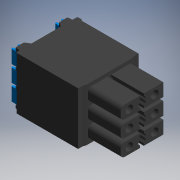
# Autodesk Inventor part: 3943136 6GD-2RR3,5-CLP-CBL
Saved by Autodesk Inventor 2017.3 (Build 213256000, 256)
## iProperties
Part Number: 3943136 6GD-2RR3,5-CLP-CBL
Material: Generic
Catalog Web Link: www.cadenas.de
Description: NEKM-C6 (p)-Terminal strip
Vendor: FESTO
Document SubType Name: Modeling
Designer: partserver
Manufacturer: FESTO
Mass: 2.36353 g
Surface Area: 19.1193 cm^2
Volume: 2.36353 cm^3
Density: 1 g/cm^3
Appearance: PSOLRGB-80-80-80
Category: PARTsolutions
Company: FESTO
Title: 3943136 6GD-2RR3,5-CLP-CBL
Author: Cadenas PARTsolutions
Comments: Terminal strip
PSOL_IDENT_0: {$CADENAS_DATA\23d-libs\festo\parts\n\nekm\parts\nekm_c6_parts.prj},197 {VTYP=3D},{NB=3943136 6GD-2R
PSOL_IDENT_1: R3,5-CLP-CBL},{LINA=3943136 6GD-2RR3,5-CLP-CBL},{NN=NEKM-C6 (p)},{DATE=16.05.2019 05:36:58},{GEOMDAT
PSOL_IDENT_2: E=16.05.2019 05:36:56},{VERSION=},{LINEID=10},{WBVAR=},{WBNUMERIC=}  {NB=3943136 6GD-2RR3,5-CLP-CBL}
PSOL_IDENT_3: ,{LINA=3943136 6GD-2RR3,5-CLP-CBL},{KT=DUMMY},{TNR=3943136},{TYP=6GD-2RR3,5-CLP-CBL},{VERS=1},{N=3},
PSOL_IDENT_4: {L=11.300},{L1=0.000}
NB: 3943136 6GD-2RR3,5-CLP-CBL
NN: NEKM-C6 (p)
NT: Terminal strip
NBSYN: $TNR. $TYP.
LINA: 3943136 6GD-2RR3,5-CLP-CBL
CATALOG: Festo
TNR: 3943136
TYP: 6GD-2RR3,5-CLP-CBL
VERS: 1
N: 3
L: 11.3
L1: 0
SUPPLIER: FESTO
ARTICLENO: 3943136 6GD-2RR3,5-CLP-CBL
BOMINFO: 3943136 6GD-2RR3,5-CLP-CBL
CREATOR: CADENAS GmbH
Autodesk Inventor part; units mm, degrees
sketch "Sketch_1" plane through (0, 0, 0) normal (0, 0, 1) x (1, 0, 0)
  line L0 (0, -4.9505) -> (0.2, -5.5)
  line L1 (0.2, -5.5) -> (0.2, -6.5)
  line L2 (0.2, -6.5) -> (13.4, -6.5)
  arc A0 (13.4, -6.5) -> (13.6, -6.3) centre (13.4, -6.3) ccw
  line L3 (13.6, -6.3) -> (13.6, 6.55)
  arc A1 (13.6, 6.55) -> (13.4, 6.75) centre (13.4, 6.55) ccw
  line L4 (13.4, 6.75) -> (12.8, 6.75)
  arc A2 (12.8, 6.75) -> (12.6, 6.55) centre (12.8, 6.55) ccw
  line L5 (12.6, 6.55) -> (12.6, 6.5)
  line L6 (12.6, 6.5) -> (0.2, 6.5)
  line L7 (0.2, 6.5) -> (0.2, 5.5)
  line L8 (0.2, 5.5) -> (0, 4.9505)
  line L9 (0, 4.9505) -> (0, -4.9505)
  constraints: 20 end point, 6 point on circle, 3 centre point
extrude "Extrusion1" add sketch "Sketch_1" along normal mid plane 11.3
sketch "Sketch_2" plane through (0, 0, 5.65) normal (0, 0, 1) x (1, 0, 0)
  line L0 (13.6, 5.85) -> (13.6, 3.0572)
  arc A0 (13.7, 3.2304) -> (13.6, 3.0572) centre (13.8, 3.0572) ccw
  line L1 (13.7, 3.2304) -> (14.5, 3.6923)
  arc A1 (14.5, 3.6923) -> (14.6, 3.8655) centre (14.4, 3.8655) ccw
  line L2 (14.6, 3.8655) -> (14.6, 5.45)
  arc A2 (14.6, 5.45) -> (14.4, 5.65) centre (14.4, 5.45) ccw
  line L3 (14.4, 5.65) -> (13.8, 5.65)
  arc A3 (13.6, 5.85) -> (13.8, 5.65) centre (13.8, 5.85) ccw
  constraints: 8 end point, 8 point on circle, 4 centre point
extrude "Extrusion2" add sketch "Sketch_2" against normal blind 0.625
sketch "Sketch_3" plane through (0, 0, 5.65) normal (0, 0, 1) x (1, 0, 0)
  arc A0 (13.8, -5.65) -> (13.6, -5.85) centre (13.8, -5.85) ccw
  line L0 (13.8, -5.65) -> (14.4, -5.65)
  arc A1 (14.4, -5.65) -> (14.6, -5.45) centre (14.4, -5.45) ccw
  line L1 (14.6, -5.45) -> (14.6, -3.8655)
  arc A2 (14.6, -3.8655) -> (14.5, -3.6923) centre (14.4, -3.8655) ccw
  line L2 (14.5, -3.6923) -> (13.7, -3.2304)
  arc A3 (13.6, -3.0572) -> (13.7, -3.2304) centre (13.8, -3.0572) ccw
  line L3 (13.6, -3.0572) -> (13.6, -5.85)
  constraints: 8 end point, 8 point on circle, 4 centre point
extrude "Extrusion3" add sketch "Sketch_3" against normal blind 0.625
pattern_linear "Rectangular Pattern1" count 2 spacing 10.675 along (0, 0, -1) of "Extrusion2"
pattern_linear "Rectangular Pattern2" count 2 spacing 10.675 along (0, 0, -1) of "Extrusion3"
sketch "Sketch_8" plane through (0, 0, 1.975) normal (0, 0, 1) x (1, 0, 0)
  line L0 (13.6, 5.85) -> (13.6, 3.0572)
  arc A0 (13.7, 3.2304) -> (13.6, 3.0572) centre (13.8, 3.0572) ccw
  line L1 (13.7, 3.2304) -> (14.5, 3.6923)
  arc A1 (14.5, 3.6923) -> (14.6, 3.8655) centre (14.4, 3.8655) ccw
  line L2 (14.6, 3.8655) -> (14.6, 5.45)
  arc A2 (14.6, 5.45) -> (14.4, 5.65) centre (14.4, 5.45) ccw
  line L3 (14.4, 5.65) -> (13.8, 5.65)
  arc A3 (13.6, 5.85) -> (13.8, 5.65) centre (13.8, 5.85) ccw
  constraints: 8 end point, 8 point on circle, 4 centre point
extrude "Extrusion4" add sketch "Sketch_8" against normal blind 0.45
pattern_linear "Rectangular Pattern3" count 2 spacing 3.5 along (0, 0, -1) of "Extrusion4"
sketch "Sketch_10" plane through (0, 0, 1.975) normal (0, 0, 1) x (1, 0, 0)
  arc A0 (13.8, -5.65) -> (13.6, -5.85) centre (13.8, -5.85) ccw
  line L0 (13.8, -5.65) -> (14.4, -5.65)
  arc A1 (14.4, -5.65) -> (14.6, -5.45) centre (14.4, -5.45) ccw
  line L1 (14.6, -5.45) -> (14.6, -3.8655)
  arc A2 (14.6, -3.8655) -> (14.5, -3.6923) centre (14.4, -3.8655) ccw
  line L2 (14.5, -3.6923) -> (13.7, -3.2304)
  arc A3 (13.6, -3.0572) -> (13.7, -3.2304) centre (13.8, -3.0572) ccw
  line L3 (13.6, -3.0572) -> (13.6, -5.85)
  constraints: 8 end point, 8 point on circle, 4 centre point
extrude "Extrusion5" add sketch "Sketch_10" against normal blind 0.45
pattern_linear "Rectangular Pattern4" count 2 spacing 3.5 along (0, 0, -1) of "Extrusion5"
sketch "Sketch_6" plane through (0, 0, 4.925) normal (0, 0, 1) x (1, 0, 0)
  line L0 (13.6, 3.85) -> (15.4, 3.85)
  arc A0 (15.4, 3.85) -> (15.6, 4.05) centre (15.4, 4.05) ccw
  line L1 (15.6, 4.05) -> (15.6, 4.0747)
  arc A1 (15.6, 4.0747) -> (15.4261, 4.273) centre (15.4, 4.0747) ccw
  line L2 (15.4261, 4.273) -> (14.4418, 4.4026)
  arc A2 (14.4418, 4.9974) -> (14.4418, 4.4026) centre (14.481, 4.7) ccw
  line L3 (14.4418, 4.9974) -> (15.4261, 5.127)
  arc A3 (15.4261, 5.127) -> (15.6, 5.3253) centre (15.4, 5.3253) ccw
  line L4 (15.6, 5.3253) -> (15.6, 5.35)
  arc A4 (15.6, 5.35) -> (15.4, 5.55) centre (15.4, 5.35) ccw
  line L5 (15.4, 5.55) -> (13.6, 5.55)
  line L6 (13.6, 5.55) -> (13.6, 3.85)
  constraints: 14 end point, 10 point on circle, 5 centre point
extrude "Extrusion6" add sketch "Sketch_6" against normal blind 2.85
pattern_linear "Rectangular Pattern5" count 3 spacing 3.5 along (0, 0, -1) count 2 spacing 9.4 along (0, -1, 0) of "Extrusion6"
sketch "Sketch_12" plane through (0, 1.8, 0) normal (0, 1, 0) x (1, 0, 0)
  line L0 (10.6, -3.5) -> (13.6, -3.5)
  line L1 (13.6, -3.5) -> (13.6, -5.2)
  arc A0 (13.6, -5.2) -> (13.4, -5) centre (13.4, -5.2) ccw
  line L2 (13.4, -5) -> (10.6, -5)
  line L3 (10.6, -5) -> (10.6, -3.5)
  line L4 (10.6, -3.5) -> (13.6, -3.5)
  constraints: 10 end point, 2 point on circle, 1 centre point
revolve "Revolution1" cut sketch "Sketch_12" angle 360 about axis through (10.6, 1.8, 3.5) along (-1, 0, 0)
pattern_linear "Rectangular Pattern6" count 3 spacing 3.5 along (0, 0, -1) count 2 spacing 3.6 along (0, -1, 0) of "Revolution1"
sketch "Sketch_14" plane through (0, 0, 0) normal (1, 0, 0) x (0, 1, 0)
  line L0 (0.4, 4.875) -> (0.4, 4.5338)
  arc A0 (0.4, 4.5338) -> (0.4586, 4.3924) centre (0.6, 4.5338) ccw
  line L1 (0.4586, 4.3924) -> (0.7278, 4.1232)
  arc A1 (0.8266, 3.777) -> (0.7278, 4.1232) centre (-0.8, 3.5) ccw
  line L2 (0.8266, 3.777) -> (0.6203, 3.5707)
  arc A2 (0.6203, 3.5707) -> (0.6203, 3.4293) centre (0.691, 3.5) ccw
  line L3 (0.6203, 3.4293) -> (0.8266, 3.223)
  arc A3 (0.7278, 2.8768) -> (0.8266, 3.223) centre (-0.8, 3.5) ccw
  line L4 (0.7278, 2.8768) -> (0.4586, 2.6076)
  arc A4 (0.4586, 2.6076) -> (0.4, 2.4662) centre (0.6, 2.4662) ccw
  line L5 (0.4, 2.4662) -> (0.4, 2.125)
  line L6 (0.4, 2.125) -> (4.6, 2.125)
  line L7 (4.6, 2.125) -> (4.6, 4.875)
  line L8 (4.6, 4.875) -> (0.4, 4.875)
  constraints: 18 end point, 10 point on circle, 5 centre point
extrude "Extrusion7" add sketch "Sketch_14" against normal blind 7.05
pattern_linear "Rectangular Pattern7" count 3 spacing 3.5 along (0, 0, -1) of "Extrusion7"
sketch "Sketch_16" plane through (0, 0, 0) normal (1, 0, 0) x (0, 1, 0)
  arc A0 (-3.6989, 4.875) -> (-4.6, 3.9739) centre (-3.6989, 3.9739) ccw
  line L0 (-4.6, 3.9739) -> (-4.6, 3.0261)
  arc A1 (-4.6, 3.0261) -> (-3.6989, 2.125) centre (-3.6989, 3.0261) ccw
  line L1 (-3.6989, 2.125) -> (-0.4, 2.125)
  line L2 (-0.4, 2.125) -> (-0.4, 2.4662)
  arc A2 (-0.4, 2.4662) -> (-0.4586, 2.6076) centre (-0.6, 2.4662) ccw
  line L3 (-0.4586, 2.6076) -> (-0.7278, 2.8768)
  arc A3 (-0.8266, 3.223) -> (-0.7278, 2.8768) centre (0.8, 3.5) ccw
  line L4 (-0.8266, 3.223) -> (-0.6203, 3.4293)
  arc A4 (-0.6203, 3.4293) -> (-0.6203, 3.5707) centre (-0.691, 3.5) ccw
  line L5 (-0.6203, 3.5707) -> (-0.8266, 3.777)
  arc A5 (-0.7278, 4.1232) -> (-0.8266, 3.777) centre (0.8, 3.5) ccw
  line L6 (-0.7278, 4.1232) -> (-0.4586, 4.3924)
  arc A6 (-0.4586, 4.3924) -> (-0.4, 4.5338) centre (-0.6, 4.5338) ccw
  line L7 (-0.4, 4.5338) -> (-0.4, 4.875)
  line L8 (-0.4, 4.875) -> (-3.6989, 4.875)
  constraints: 18 end point, 14 point on circle, 7 centre point
extrude "Extrusion8" add sketch "Sketch_16" against normal blind 7.05
pattern_linear "Rectangular Pattern8" count 3 spacing 3.5 along (0, 0, -1) of "Extrusion8"
sketch "Sketch_18" plane through (0, 2.75, 0) normal (0, 1, 0) x (1, 0, 0)
  line L0 (-6.05, -3.5) -> (-7.05, -3.5)
  line L1 (-7.05, -3.5) -> (-7.05, -2.7)
  line L2 (-7.05, -2.7) -> (-6.05, -2.7)
  line L3 (-6.05, -2.7) -> (-6.05, -3.5)
  line L4 (-6.05, -3.5) -> (-7.05, -3.5)
  constraints: 10 end point
revolve "Revolution2" cut sketch "Sketch_18" angle 360 about axis through (-6.05, 2.75, 3.5) along (1, 0, 0)
pattern_linear "Rectangular Pattern9" count 3 spacing 3.5 along (0, 0, -1) count 2 spacing 5.5 along (0, -1, 0) of "Revolution2"
ref_plane "ANBAU_XY" through (0, 0, 0) normal (0, 1, 0) x (1, 0, 0)
ref_plane "ANBAU_YZ" through (0, 0, 0) normal (1, 0, 0) x (0, 0, -1)
ref_plane "ANBAU_ZX" through (0, 0, 0) normal (0, 0, -1) x (0, 1, 0)
ref_plane "CP1_XY" through (0, 0, 0) normal (1, 0, 0) x (0, 0, -1)
ref_plane "CP1_YZ" through (0, 0, 0) normal (0, 0, -1) x (0, 1, 0)
ref_plane "CP1_ZX" through (0, 0, 0) normal (0, 1, 0) x (1, 0, 0)
body "Solid1"
